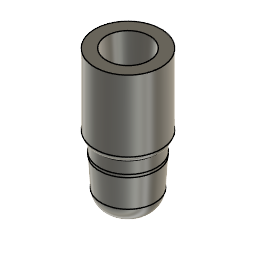
Tips Adapter (Autodesk Fusion 360 design; units mm, degrees)
part number: 2025-11-17-14-35-30-791
Autodesk Fusion 360 part; units mm, degrees
sketch "草图1" plane through (0, 0, 0) normal (0, 0, 1) x (1, 0, 0)
  circle A0 centre (0, 0) radius 2
  circle A1 centre (0, 0) radius 3
  dimension "d1" = 4
  dimension "d3" = 6
  constraint coincident A0.centre A1.centre
  measures "d1" diameter of A0
  measures "d3" diameter of A1
extrude "拉伸1" add sketch "草图1" along normal blind 8 contours A0 | A1
sketch "草图3" plane through (0, 0, 0) normal (0, 1, 0) x (1, 0, 0)
  line L0 (0, -8) -> (2.25, -8)
  line L1 (0, 0) -> (0, -8)
  line L2 (0, 0) -> (2, 0)
  line L3 (2, 0) -> (2.25, -8)
  dimension "d6" = 2.25
  constraint horizontal L0
  constraint coincident L1.start L2.start
  constraint perpendicular L0 L1
  constraint perpendicular L1 L2
  measures "d6" distance of L0.start L0.end
revolve "旋转1" cut sketch "草图3" angle 360 about axis through (0, 0, 0) along (0, 0, 1)
sketch "草图5" plane through (0, 0, 0) normal (0, 1, 0) x (1, 0, 0)
  line L0 (0, 0) -> (2.35, 0)
  line L1 (0, 0) -> (0, -5)
  line L2 (0, -5) -> (2.5, -5)
  line L3 (2.35, 0) -> (2.5, -5)
  line L4 (2.35, 0) -> (3, 0)
  line L5 (3, 0) -> (3, -5)
  line L6 (3, -5) -> (2.5, -5)
  dimension "d8" = 2.35
  dimension "d9" = 5
  constraint coincident L0.start L1.start
  constraint horizontal L0
  constraint perpendicular L0 L1
  constraint perpendicular L1 L2
  constraint parallel L0 L4
  constraint perpendicular L2 L5
  constraint perpendicular L5 L6
  measures "d8" distance of L0.start L0.end
  measures "d9" distance of L0.start L1.end
delete_face "删除面1" 1 faces at (-0.1661, -2.216, 7.1111)
extrude "拉伸2" add 1 faces at (-1.1591, 0.5829, 0) along direction (0, 0, -1) blind 4
extrude "拉伸3" add 1 faces at (-1.1591, 0.5829, -4) along direction (0, 0, -1) blind 2.5
sketch "草图7" plane through (0, 0, 0) normal (0, 1, 0) x (1, 0, 0)
  line L0 (0, -8) -> (2.25, -8)
  line L1 (0, -8) -> (0, 6.5)
  line L2 (0, 6.5) -> (1.125, 6.5)
  line L3 (1.125, 6.5) -> (2.25, -8)
  dimension "d17" = 2.25
  constraint horizontal L0
  constraint perpendicular L0 L1
  constraint perpendicular L1 L2
  measures "d17" distance of L0.start L0.end
revolve "旋转3" cut sketch "草图7" angle 360 about axis through (0, 0, 1.75) along (0, 0, 1)
sketch "草图9" plane through (0, 0, 0) normal (0, 1, 0) x (1, 0, 0)
  line L0 (0.3, 6.5) -> (0.3, 1.5)
  line L1 (0.3, 1.5) -> (3, 1.5)
  line L2 (2.7, 6.5) -> (3, 1.5)
  line L3 (2.7, 6.5) -> (3, 6.5)
  line L4 (3, 6.5) -> (3, 1.5)
  line L5 (0.3, 6.5) -> (2.5, 6.5)
  dimension "d20" = 2.4
  dimension "d21" = 5
  constraint perpendicular L0 L1
  constraint coincident L3 L5.end
  constraint perpendicular L0 L5
  measures "d20" distance of L0.start L2.start
  measures "d21" distance of L0.start L0.end
sketch "草图10" plane through (0, 0, 0) normal (0, 1, 0) x (1, 0, 0)
revolve "旋转4" cut sketch "草图9" angle 360 about axis through (0, 0, 1.75) along (0, 0, 1)
fillet "圆角2" radius 4 1 edges at (-2.797, -1.0848, -1.5)
delete_face "删除面2" 1 faces at (2.9837, -0.2986, -1.4866)
fillet "圆角3" radius 0.75 1 edges at (-2.5173, 0.9764, -6.5)
fillet "圆角4" radius 5 1 edges at (-2.797, 1.0848, -1.5)
sketch "草图11" plane through (0, 0, 8) normal (0, 0, 1) x (-1, 0, 0)
  circle A0 centre (0, 0) radius 2.25
  circle A1 centre (0, 0) radius 3
  circle A2 centre (0, 0) radius 3.47
  constraint coincident A0.centre A1.centre
extrude "拉伸4" add sketch "草图11" against normal blind 8.1 contours A2
fillet "圆角5" radius 0.7 1 edges at (3.2352, -1.2548, -0.1)
delete_face "删除面3" 1 faces at (2.7081, -0.271, -5.9305)
fillet "圆角6" radius 2 1 edges at (-2.5173, -0.9764, -6.5)
